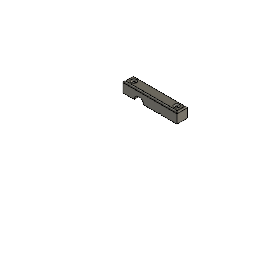
cable_clamp v1 (Autodesk Fusion 360 design; units mm, degrees)
Autodesk Fusion 360 part; units mm, degrees
sketch "Sketch1" plane through (0, 0, 36) normal (0, 0, 1) x (-1, 0, 0)
  line L0 (-64.8, -3) -> (-106, -3)
  line L1 (-106, -3) -> (-106, -11)
  line L2 (-106, -11) -> (-64.8, -11)
  line L3 (-64.8, -11) -> (-64.8, -3)
  circle A0 centre (-69.15, -7) radius 1
  circle A1 centre (-101.65, -7) radius 1
  dimension "d1" = 2
  dimension "d2" = 4.35
  dimension "d3" = 4
  dimension "d4" = 2
  dimension "d5" = 4.35
  dimension "d6" = 4
  measures "d1" diameter of A0
  measures "d2" distance of L3 A0.centre
  measures "d3" distance of L2 A0.centre
  measures "d4" diameter of A1
  measures "d5" distance of L1 A1.centre
  measures "d6" distance of L2 A1.centre
sketch "Sketch2" plane through (0, 11, 0) normal (0, 1, 0) x (-1, 0, 0)
  arc A0 (-93.75, 28) -> (-92.25, 28) centre (-93, 28) ccw
  line L0 (-93.75, 28) -> (-106, 28)
  line L1 (-106, 28) -> (-106, 23)
  line L2 (-106, 23) -> (-94, 23)
  line L3 (-94, 23) -> (-94, 3)
  line L4 (-94, 3) -> (-64.8, 3)
  line L5 (-64.8, 3) -> (-64.8, 28)
  line L6 (-64.8, 28) -> (-73.5, 28)
  arc A1 (-80.5, 28) -> (-73.5, 28) centre (-77, 28) ccw
  line L7 (-80.5, 28) -> (-92.25, 28)
  line L8 (-64.8, 28) -> (-64.8, 36)
  line L9 (-64.8, 36) -> (-106, 36)
  line L10 (-106, 36) -> (-106, 28)
  arc A2 (-73.5, 28) -> (-80.5, 28) centre (-77, 28) ccw
  arc A3 (-92.25, 28) -> (-93.75, 28) centre (-93, 28) ccw
  line L11 (-106, 28) -> (-93.75, 28)
  line L12 (-92.25, 28) -> (-80.5, 28)
  line L13 (-73.5, 28) -> (-64.8, 28)
  dimension "d7" = 8
  dimension "d8" = 41.2
  dimension "d9" = 7
  dimension "d10" = 1.5
  constraint horizontal L11
  constraint vertical L8
  constraint horizontal L9
  constraint vertical L10
  constraint coincident L0.end L1.start
  constraint concentric A1 A2
  constraint concentric A0 A3
  constraint collinear L11 L12
  constraint collinear L12 L13
  measures "d7" distance of L0.end L9.end
  measures "d8" distance of L8.end L9.end
  measures "d9" diameter of A2
  measures "d10" diameter of A3
extrude "Extrude1" add sketch "Sketch2" against normal up to surface (8 mm away) contours L0 L6 L7 L8 L9 L10 A2 A3 L11 L12 L13
extrude "Extrude2" cut sketch "Sketch1" against normal up to surface (8 mm away) contours A0 | A1
fillet "Fillet1" radius 1 6 edges at (102.5823, 6.6384, 36) (70.0823, 6.6384, 36) (106, 7, 36) (85.4, 11, 36) (64.8, 7, 36) (85.4, 3, 36)
